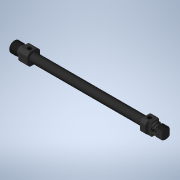
# Autodesk Inventor part: 19182 DSNU-8-100-P---(A----0-ZR)
Saved by Autodesk Inventor 2021 (Build 250183000, 183)
## iProperties
Created: 2026-04-16
Part Number: 19182 DSNU-8-100-P---(A----0-ZR)
Material: Generic
Catalog Web Link: www.3dfindit.com
Description: DSNU---(ZR)-ISO cylinder
Vendor: FESTO
Document SubType Name: Modeling
Designer: psAdmin
Manufacturer: FESTO
Mass: 8.3553 g
Surface Area: 94.0648 cm^2
Volume: 8.3553 cm^3
Density: 1 g/cm^3
Appearance: PSOLRGB-176-176-176
Category: PARTsolutions
Company: FESTO
Title: 19182 DSNU-8-100-PA--0--
Author: Cadenas PARTsolutions
Comments: ISO cylinder
PSOL_IDENT_0: {$CADENAS_DATA/23d-libs/festo/parts/d/dsnu/parts/dsnu_metric_zr.prj},241 {VTYP=3D},{NB=19182 DSNU-8-
PSOL_IDENT_1: 100-P---(A----0-ZR)},{LINA=19182 DSNU-8-100-PA--0--},{NN=DSNU---(ZR)},{DATE=03.04.2026 17:15:03},{GE
PSOL_IDENT_2: OMDATE=26.03.2026 09:11:34},{VERSION=},{LINEID=10},{WBVAR=TNR,HUB,DA,PE,ZD,VS,KA,HE,K8,KP,R8},{WBNUM
PSOL_IDENT_3: ERIC=HUB,K8}  {NB=19182 DSNU-8-100-P---(A----0-ZR)},{LINA=19182 DSNU-8-100-PA--0--},{KT=DUMMY},{TNR=
PSOL_IDENT_4: 19182},{TYP=DSNU-8},{DSNU=METRIC},{DE=D},{KDM=8},{HUB=100},{DA=P},{DA1='P'},{PE=A},{ZD=-},{VS=-},{VS
PSOL_IDENT_5: ALG='-'},{KA=-},{KAALG='-','S2'},{HE=-},{HE1='-','15KE'},{HET=},{K8=0},{KP=-},{KPALG='-','KP'},{R8=-
PSOL_IDENT_6: },{R81='-'},{R8H=0.000},{A1=15},{A2=50},{A3=4},{A4=29.0},{AB=12},{AM=12},{B=12},{BB=3},{BE=M12x1,25}
PSOL_IDENT_7: ,{BENDM=12.000},{BEKDM=10.466},{BEP=1.250},{BS=3.4},{B1=24},{B2=0},{B3=0},{B4=0},{B5=14.0},{B6=6},{B
PSOL_IDENT_8: 7=0},{CD=4},{D=16},{D10=15},{D20=16},{D1=12},{D2=4},{D3=9.3},{D4=0.0},{D5=10.5},{D6=0},{D7=0},{EE=M5
PSOL_IDENT_9: },{EENDM=5.0000},{EEKDM=4.0190},{EW=8},{F=18},{FF=M3},{FFNDM=3.000},{FFKDM=2.387},{F1=0},{H=16},{H1=
PSOL_IDENT_10: 0},{KK=M4},{KKNDM=4.0000},{KKKDM=3.1410},{KKP=0.000},{K1=-},{K1NDM=0.000},{K1KDM=0.000},{K2=0.0},{KV=
PSOL_IDENT_11: 19},{KW=6},{L=6},{LH=5.0},{LK=7.6},{L1=74},{L2=46},{L3=6.0},{L4=12.0},{L5=10},{L6=28},{L7=16},{L8=10
PSOL_IDENT_12: .0},{L9=16.0},{L10=53.7},{L11=61.7},{L12=43.6},{L13=78.0},{ST=3.4},{SW=0},{T=0},{WH=16},{X=0.0},{XC=
PSOL_IDENT_13: 64},{K1KP=27},{K2KP=M5},{K2KPNDM=5.000},{K3KP=11},{K4KP=13.5},{K5KP=34.5},{K6KP=4.2},{K7KP=12},{K8KP=
PSOL_IDENT_14: 19.5},{K9KP=8.0},{K10KP=0.0},{K11KP=0},{K12KP=M5},{K12KPNDM=5.000},{K13KP=29.000},{ZRSTART=22},{MHL=
PSOL_IDENT_15: 17.700},{ZRL=26},{C=14.000},{C1=9.500},{C2=14.000},{WHX=8.000},{LD1=10.300},{LD2=10.000},{AD1=7.000}
PSOL_IDENT_16: ,{AD2=5.000},{AD3=8.000},{AD4=6.000},{AD5=0.000},{MH1=6.000},{MH2=2.400},{MH3=8.000},{KP1=16.000},{K
PSOL_IDENT_17: P2=9.500},{KP3=7.000},{KP4=12.000},{KP5=16.000},{KPC=10.000},{KPF=2.000},{KPG=7.000},{KPH=28.000},{K
PSOL_IDENT_18: PJ=11.500},{KPK=10.500},{KPL=1.500},{KPR3=0.400},{KPR=11.000},{KPS=6.000},{MLD1=25.000},{MLD2=20.000
PSOL_IDENT_19: },{MLD3=3.000},{MLL1=8.000},{PPVSTD=0.000},{PPVMH=0.000},{PPVMQ=0.000},{PPVY=0.000},{PPVZ=0.000},{PP
PSOL_IDENT_20: VZ1=0.000},{PPVZ2=0.000},{PPVA=0.000},{PPVB=0.000},{PPVC=0.000},{PPVD=0.000},{PPVE=0.000},{PPVE1=0.0
PSOL_IDENT_21: 00},{PPVE2=0.000},{PPVH=0.000},{KL1=35.5},{SWL=0.000},{K3L=0.000},{ES1=1.000},{ES2=0.000},{KPVERS=0}
PSOL_IDENT_22: ,{HUB1=100},{NUTOFF=8.000},{DIMZJREAR=170},{KAVERS=0},{VERS=2},{H2=0},{GLD=5.000},{GLL=8.000}
NB: 19182 DSNU-8-100-P---(A----0-ZR)
NN: DSNU---(ZR)
NT: ISO cylinder
NBSYN: $TNR. $TYP.-$HUB1.-$DA.---($PE.$ZD.$VS.$KA.$HET.$KP.$K8.$R8.ZR)
LINA: 19182 DSNU-8-100-PA--0--
CATALOG: Festo
TNR: 19182
TYP: DSNU-8
DSNU: METRIC
DE: D
KDM: 8
HUB: 100
DA: P
DA1: 'P'
PE: A
ZD: -
VS: -
KA: -
HE: -
K8: 0
KP: -
R8: -
R81: '-'
R8H: 0
A1: 15
A2: 50
A3: 4
A4: 29
AB: 12
AM: 12
B: 12
BB: 3
BE: M12x1,25
BENDM: 12
BEKDM: 10.466
BEP: 1.25
BS: 3.4
B1: 24
B2: 0
B3: 0
B4: 0
B5: 14
B6: 6
B7: 0
CD: 4
D10: 15
D20: 16
D1: 12
D2: 4
D3: 9.3
D4: 0
D5: 10.5
D6: 0
D7: 0
EE: M5
EENDM: 5
EEKDM: 4.019
EW: 8
F: 18
FF: M3
FFNDM: 3
FFKDM: 2.387
F1: 0
H: 16
H1: 0
KK: M4
KKNDM: 4
KKKDM: 3.141
KKP: 0
K1: -
K1NDM: 0
K1KDM: 0
K2: 0
KV: 19
KW: 6
L: 6
LH: 5
LK: 7.6
L3: 6
L4: 12
L5: 10
L6: 28
L7: 16
L8: 10
L9: 16
L13: 78
ST: 3.4
SW: 0
T: 0
X: 0
K1KP: 27
K2KP: M5
K2KPNDM: 5
K3KP: 11
K4KP: 13.5
K5KP: 34.5
K6KP: 4.2
K7KP: 12
K8KP: 19.5
K9KP: 8
K10KP: 0
K11KP: 0
K12KP: M5
K12KPNDM: 5
K13KP: 29
MHL: 17.7
C1: 9.5
C2: 14
WHX: 8
LD1: 10.3
LD2: 10
AD1: 7
AD2: 5
AD3: 8
AD4: 6
AD5: 0
MH1: 6
MH2: 2.4
MH3: 8
KP1: 16
KP2: 9.5
KP3: 7
KP4: 12
KP5: 16
KPC: 10
KPF: 2
KPG: 7
KPH: 28
KPJ: 11.5
KPK: 10.5
KPL: 1.5
KPR3: 0.4
KPR: 11
KPS: 6
MLD1: 25
MLD2: 20
MLD3: 3
MLL1: 8
PPVSTD: 0
PPVMH: 0
PPVMQ: 0
PPVY: 0
PPVZ1: 0
PPVZ2: 0
PPVA: 0
PPVB: 0
PPVC: 0
PPVD: 0
PPVE1: 0
PPVE2: 0
PPVH: 0
SWL: 0
K3L: 0
ES1: 1
ES2: 0
NUTOFF: 8
H2: 0
GLD: 5
GLL: 8
SUPPLIER: FESTO
ARTICLENO: 19182 DSNU-8-100-P---(A----0-ZR)
BOMINFO: 19182 DSNU-8-100-PA--0--
CREATOR: CADENAS GmbH
Autodesk Inventor part; units mm, degrees
sketch "Sketch_1" plane through (0, 0, 0) normal (0, 0, 1) x (1, 0, 0)
  line L0 (12, 0) -> (0, 0)
  line L1 (0, 0) -> (0, 5.15)
  line L2 (0, 5.15) -> (0.85, 6)
  line L3 (0.85, 6) -> (7.35, 6)
  line L4 (7.35, 6) -> (8.1743, 5.1757)
  arc A0 (8.1743, 5.1757) -> (8.5985, 5) centre (8.5985, 5.6) ccw
  line L5 (8.5985, 5) -> (9.4, 5)
  arc A1 (9.4, 5) -> (10, 5.6) centre (9.4, 5.6) ccw
  line L6 (10, 5.6) -> (10, 6)
  line L7 (10, 6) -> (12, 6)
  line L8 (12, 6) -> (12, 0)
  line L9 (12, 0) -> (0, 0)
  constraints: 20 end point, 4 point on circle, 2 centre point
revolve "Revolution1" add sketch "Sketch_1" angle 360 about axis through (12, 0, 0) along (1, 0, 0)
thread "Thread1" size "M12x1.25" class "6g" standard "ISO Metric profile" full length
sketch "Sketch_2" plane through (12, 0, 0) normal (1, 0, 0) x (0, 0, -1)
  arc A0 (-7, -3.873) -> (-3.873, -7) centre (0, 0) ccw
  line L0 (-3.873, -7) -> (3.873, -7)
  arc A1 (3.873, -7) -> (7, -3.873) centre (0, 0) ccw
  line L1 (7, -3.873) -> (7, 3.873)
  arc A2 (7, 3.873) -> (3.873, 7) centre (0, 0) ccw
  line L2 (3.873, 7) -> (-3.873, 7)
  arc A3 (-3.873, 7) -> (-7, 3.873) centre (0, 0) ccw
  line L3 (-7, 3.873) -> (-7, -3.873)
  constraints: 8 end point, 8 point on circle, 4 centre point
extrude "Extrusion1" add sketch "Sketch_2" along normal blind 10
sketch "Sketch_3" plane through (0, 0, 0) normal (0, 0, 1) x (1, 0, 0)
  line L0 (148, 0) -> (22, 0)
  line L1 (22, 0) -> (22, 4.65)
  line L2 (22, 4.65) -> (148, 4.65)
  line L3 (148, 4.65) -> (148, 0)
  line L4 (148, 0) -> (22, 0)
  constraints: 10 end point
revolve "Revolution2" add sketch "Sketch_3" angle 360 about axis through (148, 0, 0) along (1, 0, 0)
sketch "Sketch_16" plane through (148, 0, 0) normal (1, 0, 0) x (0, 0, -1)
  line L0 (-7, -7) -> (7, -7)
  line L1 (7, -7) -> (7, 7)
  line L2 (7, 7) -> (-7, 7)
  line L3 (-7, 7) -> (-7, -7)
  constraints: 8 end point
extrude "Extrusion2" add sketch "Sketch_16" along normal blind 10
sketch "Sketch_124" plane through (0, 0, 0) normal (0, 0, 1) x (1, 0, 0)
  line L0 (158, 0) -> (148, 0)
  line L1 (148, 18) -> (148, 8)
  line L2 (148, 8) -> (158, 8)
  line L3 (158, 8) -> (158, 18)
  line L4 (158, 18) -> (148, 18)
  constraints: 10 end point
revolve "Revolution3" cut sketch "Sketch_124" angle 360 about axis through (158, 0, 0) along (1, 0, 0)
sketch "Sketch_23" plane through (0, 0, 0) normal (0, 0, 1) x (1, 0, 0)
  line L0 (170, 0) -> (158, 0)
  line L1 (158, 0) -> (158, 6)
  line L2 (158, 6) -> (160, 6)
  line L3 (160, 6) -> (160, 5.6)
  arc A0 (160, 5.6) -> (160.6, 5) centre (160.6, 5.6) ccw
  line L4 (160.6, 5) -> (161.4015, 5)
  arc A1 (161.4015, 5) -> (161.8257, 5.1757) centre (161.4015, 5.6) ccw
  line L5 (161.8257, 5.1757) -> (162.65, 6)
  line L6 (162.65, 6) -> (169.15, 6)
  line L7 (169.15, 6) -> (170, 5.15)
  line L8 (170, 5.15) -> (170, 0)
  line L9 (170, 0) -> (158, 0)
  constraints: 20 end point, 4 point on circle, 2 centre point
revolve "Revolution4" add sketch "Sketch_23" angle 360 about axis through (170, 0, 0) along (1, 0, 0)
thread "Thread2" size "M12x1.25" class "6g" standard "ISO Metric profile" full length
sketch "Sketch_6" plane through (0, 0, 0) normal (0, 1, 0) x (-1, 0, 0)
  line L0 (-154, -12) -> (-154, -4)
  line L1 (-154, -4) -> (-170, -4)
  line L2 (-170, -4) -> (-170, 4)
  line L3 (-170, 4) -> (-154, 4)
  line L4 (-154, 4) -> (-154, 12)
  line L5 (-154, 12) -> (-178, 12)
  line L6 (-178, 12) -> (-178, -12)
  line L7 (-178, -12) -> (-154, -12)
  constraints: 16 end point
extrude "Extrusion3" cut sketch "Sketch_6" along normal mid plane 16
sketch "Sketch_147" plane through (160, 0, 0) normal (1, 0, 0) x (0, 0, -1)
  line L0 (4, 0) -> (-4.2, 0)
  line L1 (-4.2, 0) -> (-4.2, 3.1928)
  line L2 (-4.2, 3.1928) -> (-3, 2.5)
  line L3 (-3, 2.5) -> (-3.5, 2.5)
  line L4 (-3.5, 2.5) -> (-4, 2.2113)
  line L5 (-4, 2.2113) -> (-4, 2)
  line L6 (-4, 2) -> (4, 2)
  line L7 (4, 2) -> (4, 2.2113)
  line L8 (4, 2.2113) -> (3.5, 2.5)
  line L9 (3.5, 2.5) -> (3, 2.5)
  line L10 (3, 2.5) -> (4.2, 3.1928)
  line L11 (4.2, 3.1928) -> (4.2, 0)
  line L12 (4.2, 0) -> (-4.2, 0)
  constraints: 26 end point
revolve "Revolution5" cut sketch "Sketch_147" angle 360 about axis through (160, 0, -4) along (0, 0, -1)
sketch "Sketch9" plane through (12, 7, 3.873) normal (0, 1, 0) x (1, 0, 0)
  point P0 (6, 3.873)
hole "Hole1" at (18, 7, 0) direction (0, -1, 0) diameter 4.134 depth 7 countersink diameter 5 countersink angle 90 thread size "M5x0.8" class "6H" standard "ISO Metric profile"
sketch "Sketch10" plane through (148, 7, 3.873) normal (0, 1, 0) x (1, 0, 0)
  point P0 (4, 3.873)
hole "Hole2" at (152, 7, 0) direction (0, -1, 0) diameter 4.134 depth 8 tip angle 120 countersink diameter 5 countersink angle 90 thread size "M5x0.8" class "6H" standard "ISO Metric profile"
sketch "Sketch_64" plane through (0, 0, 0) normal (0, 0, 1) x (1, 0, 0)
  line L0 (133.5, 0) -> (-4, 0)
  line L1 (-4, 0) -> (-4, 2)
  line L2 (-4, 2) -> (31.5, 2)
  line L3 (31.5, 2) -> (31.5, 4)
  line L4 (31.5, 4) -> (133.5, 4)
  line L5 (133.5, 4) -> (133.5, 0)
  line L6 (133.5, 0) -> (-4, 0)
  constraints: 14 end point
revolve "Revolution6" cut sketch "Sketch_64" angle 360 about axis through (133.5, 0, 0) along (1, 0, 0)
ref_plane "FDT_FRONT_XY" through (12, 0, 0) normal (1, 0, 0) x (0, 0, -1)
ref_plane "FDT_FRONT_YZ" through (12, 0, 0) normal (0, 0, -1) x (0, 1, 0)
ref_plane "FDT_FRONT_ZX" through (12, 0, 0) normal (0, 1, 0) x (1, 0, 0)
ref_plane "FDT_QSFRONT_XY" through (18, 7, 0) normal (0, 1, 0) x (0, 0, 1)
ref_plane "FDT_QSFRONT_YZ" through (18, 7, 0) normal (0, 0, 1) x (1, 0, 0)
ref_plane "FDT_QSFRONT_ZX" through (18, 7, 0) normal (1, 0, 0) x (0, 1, 0)
ref_plane "FDT_QSREAR_XY" through (152, 7, 0) normal (0, 1, 0) x (0, 0, 1)
ref_plane "FDT_QSREAR_YZ" through (152, 7, 0) normal (0, 0, 1) x (1, 0, 0)
ref_plane "FDT_QSREAR_ZX" through (152, 7, 0) normal (1, 0, 0) x (0, 1, 0)
ref_plane "FDT_REAR_XY" through (158, 0, 0) normal (-1, 0, 0) x (0, 0, -1)
ref_plane "FDT_REAR_YZ" through (158, 0, 0) normal (0, 0, -1) x (0, -1, 0)
ref_plane "FDT_REAR_ZX" through (158, 0, 0) normal (0, -1, 0) x (-1, 0, 0)
ref_plane "FDT_SMBR1_XY" through (31.5, 0, 0) normal (-1, 0, 0) x (0, 0, 1)
ref_plane "FDT_SMBR1_YZ" through (31.5, 0, 0) normal (0, 0, 1) x (0, 1, 0)
ref_plane "FDT_SMBR1_ZX" through (31.5, 0, 0) normal (0, 1, 0) x (-1, 0, 0)
ref_plane "FDT_SMBR2_XY" through (138.5, 0, 0) normal (-1, 0, 0) x (0, 0, 1)
ref_plane "FDT_SMBR2_YZ" through (138.5, 0, 0) normal (0, 0, 1) x (0, 1, 0)
ref_plane "FDT_SMBR2_ZX" through (138.5, 0, 0) normal (0, 1, 0) x (-1, 0, 0)
ref_plane "FDT_SWIVELAXIS_XY" through (160, 0, 0) normal (0, 0, 1) x (1, 0, 0)
ref_plane "FDT_SWIVELAXIS_YZ" through (160, 0, 0) normal (1, 0, 0) x (0, 1, 0)
ref_plane "FDT_SWIVELAXIS_ZX" through (160, 0, 0) normal (0, 1, 0) x (0, 0, 1)
ref_plane "NUT_XY" through (6, 0, 0) normal (1, 0, 0) x (0, 0, -1)
ref_plane "NUT_YZ" through (6, 0, 0) normal (0, 0, -1) x (0, 1, 0)
ref_plane "NUT_ZX" through (6, 0, 0) normal (0, 1, 0) x (1, 0, 0)
ref_plane "ZR_XY" through (0, 0, 0) normal (-1, 0, 0) x (0, 0, -1)
ref_plane "ZR_YZ" through (0, 0, 0) normal (0, 0, -1) x (0, -1, 0)
ref_plane "ZR_ZX" through (0, 0, 0) normal (0, -1, 0) x (-1, 0, 0)
ref_plane "ZYL_XY" through (12, 0, 0) normal (1, 0, 0) x (0, 0, -1)
ref_plane "ZYL_YZ" through (12, 0, 0) normal (0, 0, -1) x (0, 1, 0)
ref_plane "ZYL_ZX" through (12, 0, 0) normal (0, 1, 0) x (1, 0, 0)
body "Solid1"
